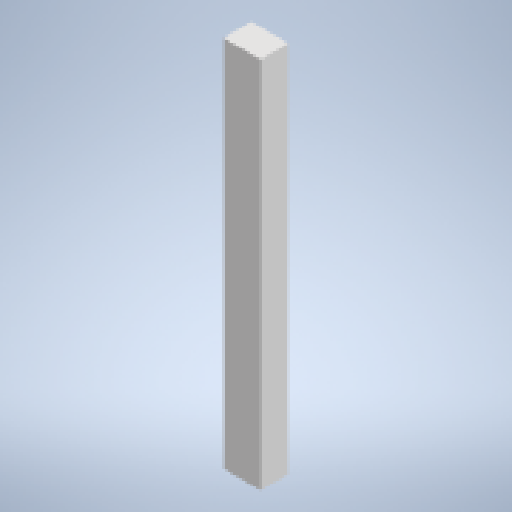
# Autodesk Inventor part: guide corte y
Saved by Autodesk Inventor 2024 (Build 280153000, 153)
## iProperties
Created: 2023-12-23
Part Number: guide corte y
Material: Generico
Document SubType Name: Modeling
Designer: Giorgio
Density: 1 g/cm^3
Appearance: Default
Mass: 77.7035 g
Surface Area: 213.04 cm^2
Volume: 77.7035 cm^3
Author: Giorgio
Autodesk Inventor part; units mm, degrees
ref_plane "YZ Plane" through (0, 0, 0) normal (1, 0, 0) x (0, 1, 0)
ref_plane "XZ Plane" through (0, 0, 0) normal (0, 1, 0) x (-1, 0, 0)
ref_plane "XY Plane" through (0, 0, 0) normal (0, 0, 1) x (1, 0, 0)
sketch "Schizzo1" plane through (0, 0, 0) normal (0, 0, 1) x (1, 0, 0)
  line L0 (47.7569, 145.2967) -> (7.7569, 145.2967)
  line L1 (7.7569, 145.2967) -> (7.7569, -254.7033)
  line L2 (7.7569, -254.7033) -> (47.7569, -254.7033)
  line L3 (47.7569, -254.7033) -> (47.7569, 145.2967)
  point P0 (0, 0)
  dimension "d0" = 400
  dimension "d1" = 40
  constraints: 8 end point, 2 parallel, 1 horizontal, 1 perpendicular
  measures "d0" distance of L2.end L0.start
  measures "d1" distance of L1.end L2.end
extrude "Estrusione1" add sketch "Schizzo1" along normal blind 30
